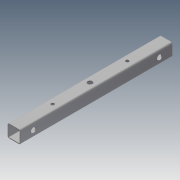
# Autodesk Inventor part: feed-bpsupxp
Saved by Autodesk Inventor 2013 SP2 (Build 170200200, 200)
## iProperties
Company: HERA Project
Created: 2013-06-27
Part Number: feed-bpsupxp
Material: Steel
Description: Feed backplane support crosspiece
Document SubType Name: Modeling
Designer: Dave
Mass: 413.229 g
Surface Area: 640.686 cm^2
Volume: 52.6407 cm^3
Density: 7.85 g/cm^3
Title: feed-bpsupxp
Author: David DeBoer
Autodesk Inventor part; units mm, degrees
ref_plane "YZ Plane" through (0, 0, 0) normal (1, 0, 0) x (0, 1, 0)
ref_plane "XZ Plane" through (0, 0, 0) normal (0, 1, 0) x (-1, 0, 0)
ref_plane "XY Plane" through (0, 0, 0) normal (0, 0, 1) x (1, 0, 0)
sketch "Sketch1" plane through (0, 0, 0) normal (0, 0, 1) x (1, 0, 0)
  line L0 (3.175, 0) -> (22.225, 0)
  line L1 (25.4, 3.175) -> (25.4, 22.225)
  line L2 (22.225, 25.4) -> (3.175, 25.4)
  line L3 (0, 22.225) -> (0, 3.175)
  arc A0 (3.175, 25.4) -> (0, 22.225) centre (3.175, 22.225) ccw
  arc A1 (0, 3.175) -> (3.175, 0) centre (3.175, 3.175) ccw
  arc A2 (22.225, 0) -> (25.4, 3.175) centre (22.225, 3.175) ccw
  arc A3 (25.4, 22.225) -> (22.225, 25.4) centre (22.225, 22.225) ccw
  line L4 (3.175, 23.749) -> (22.225, 23.749)
  arc A4 (23.749, 22.225) -> (22.225, 23.749) centre (22.225, 22.225) ccw
  line L5 (23.749, 22.225) -> (23.749, 3.175)
  arc A5 (22.225, 1.651) -> (23.749, 3.175) centre (22.225, 3.175) ccw
  line L6 (22.225, 1.651) -> (3.175, 1.651)
  arc A6 (1.651, 3.175) -> (3.175, 1.651) centre (3.175, 3.175) ccw
  line L7 (1.651, 3.175) -> (1.651, 22.225)
  arc A7 (3.175, 23.749) -> (1.651, 22.225) centre (3.175, 22.225) ccw
  point P0 (0, 0)
  point P1 (25.4, 0)
  point P2 (0, 25.4)
  dimension "d0" = 25.4
  dimension "d1" = 25.4
  dimension "d2" = 3.175
  dimension "d3" = 1.651
  constraints: 16 end point, 16 point on circle, 8 centre point, 8 tangent, 6 point on line, 4 parallel, 3 equal radius, 2 perpendicular, 1 horizontal, 7 other
  measures "d0" distance of point (0, 0) point (25.4, 0)
  measures "d1" distance of point (0, 25.4) point (0, 0)
  measures "d2" radius of A0
  measures "d3" distance between parallel lines of L4 L2
extrude "Extrusion1" add sketch "Sketch1" along normal blind 299.72
sketch "Sketch2" plane through (3.175, 25.4, 0) normal (0, 1, 0) x (1, 0, 0)
  line L0 (0, 0) -> (0, -299.72) projected
  line L1 (19.05, 0) -> (19.05, -299.72) projected
  line L2 (0, -149.86) -> (19.05, -149.86) construction
  circle A0 centre (9.525, -149.86) radius 3.175
  point P0 (-3.175, 0)
  dimension "d6" = 6.35
  constraints: 3 midpoint, 2 end point, 1 centre point
  measures "d6" diameter of A0
hole "Hole1" at (12.7, 25.4, 149.86) direction (0, -1, 0) diameter 9.525 end through all
sketch "Sketch3" plane through (3.175, 25.4, 0) normal (0, 1, 0) x (1, 0, 0)
  circle A0 centre (9.525, -149.86) radius 4.7625 projected
  line L0 (19.05, 0) -> (0, 0) projected
  line L1 (19.05, -299.72) -> (0, -299.72) projected
  line L2 (19.05, 0) -> (19.05, -299.72) projected
  line L3 (9.525, 0) -> (9.525, -299.72) construction
  circle A1 centre (9.525, -76.2) radius 2.6066
  line L4 (9.525, -149.86) -> (19.05, -149.86) construction
  circle A2 centre (9.525, -223.52) radius 2.6066
  point P0 (-3.175, 0)
  dimension "d14" = 76.2
  constraints: 4 end point, 3 midpoint, 2 centre point, 1 point on line, 1 symmetric about line, 1 other
  measures "d14" distance from line of A1.centre L0
hole "Hole2" at (12.7, 25.4, 76.2) at (12.7, 25.4, 223.52) direction (0, -1, 0) diameter 6.35 end through all
sketch "Sketch4" plane through (25.4, 3.175, 0) normal (1, 0, 0) x (0, 0, -1)
  line L0 (0, 19.05) -> (-299.72, 19.05) projected
  line L1 (-299.72, 0) -> (-299.72, 19.05) projected
  line L2 (0, 0) -> (-299.72, 0) projected
  circle A0 centre (-274.32, 9.525) radius 3.2646
  line L3 (-149.86, 19.05) -> (-149.86, 0) construction
  point P0 (0, -3.175)
  dimension "d22" = 25.4
  constraints: 2 end point, 2 midpoint, 1 centre point
  measures "d22" distance from line of A0.centre L1
hole "Hole3" at (25.4, 12.7, 274.32) direction (-1, 0, 0) diameter 9.525 end through all
sketch "Sketch6" plane through (3.175, 0, 0) normal (0, -1, 0) x (1, 0, 0)
  circle A0 centre (9.525, 223.52) radius 3.175 projected
  circle A1 centre (9.525, 149.86) radius 4.7625 projected
  line L0 (19.05, 0) -> (19.05, 299.72) projected
  line L1 (0, 0) -> (0, 299.72) projected
  line L2 (9.525, 223.52) -> (9.525, 149.86) construction
  line L3 (9.525, 149.86) -> (19.05, 149.86) construction
  circle A2 centre (9.525, 187.96) radius 3.6104
  circle A3 centre (9.525, 111.76) radius 3.6104
  point P0 (-3.175, 0)
  dimension "d32" = 35.56
  dimension "d33" = 76.2
  constraints: 4 end point, 2 centre point, 1 midpoint, 1 parallel, 1 point on line, 1 symmetric about line, 1 other
  measures "d32" distance of A2.centre L2.start
  measures "d33" distance of A3.centre A2.centre
hole "Hole4" at (12.7, 0, 187.96) at (12.7, 0, 111.76) direction (0, 1, 0) diameter 3.9624 depth 16.51 tip angle 118 thread size "10-32 UNF" class "2B" standard "ANSI Unified Screw Threads"
sketch "Sketch7" plane through (25.4, 3.175, 0) normal (1, 0, 0) x (0, 0, -1)
  line L0 (0, 0) -> (0, 19.05) projected
  circle A0 centre (-25.4, 9.525) radius 3.0513
  point P0 (0, -3.175)
  dimension "d41" = 25.4
  constraints: 1 centre point
  measures "d41" distance from line of A0.centre L0
hole "Hole5" at (25.4, 12.7, 25.4) direction (-1, 0, 0) diameter 9.525 end through all
body "Solid1"
